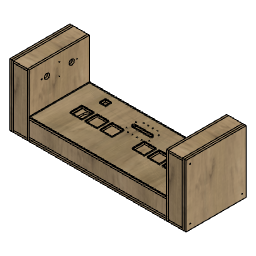
ongekicon-diy (Autodesk Fusion 360 design; units mm, degrees)
Autodesk Fusion 360 part; units mm, degrees
sketch "스케치1" plane through (0, 0, 0) normal (0, 0, 1) x (1, 0, 0)
  line L0 (289, -642.7336) -> (375, -642.7336)
  line L1 (375, -656.7336) -> (289, -656.7336)
  arc A0 (289, -642.7336) -> (289, -656.7336) centre (289, -649.7336) ccw
  arc A1 (375, -656.7336) -> (375, -642.7336) centre (375, -649.7336) ccw
  arc A2 (375, -656.7336) -> (375, -642.7336) centre (375, -649.7336) ccw
  circle A3 centre (277.0783, -626.5501) radius 2.65
  circle A4 centre (277.0783, -672.9171) radius 2.65
  circle A5 centre (386.9217, -626.4866) radius 2.65
  circle A6 centre (386.9217, -672.8535) radius 2.65
  circle A7 centre (299.0783, -611.6097) radius 2.65
  circle A8 centre (321.0783, -611.6097) radius 2.65
  circle A9 centre (343.0783, -611.6097) radius 2.65
  circle A10 centre (365.0783, -611.6097) radius 2.65
  circle A11 centre (364.9217, -687.7939) radius 2.65
  circle A12 centre (342.9217, -687.7939) radius 2.65
  circle A13 centre (320.9217, -687.7939) radius 2.65
  circle A14 centre (298.9217, -687.7939) radius 2.65
  line L2 (0, -575) -> (664, -575)
  line L3 (664, -575) -> (664, -866)
  line L4 (664, -866) -> (0, -866)
  line L5 (0, -866) -> (0, -575)
  line L6 (0, -1260) -> (664, -1260)
  line L7 (664, -1260) -> (664, -1333)
  line L8 (664, -1333) -> (0, -1333)
  line L9 (0, -1333) -> (0, -1260)
  line L10 (0, -1495) -> (0, -1422)
  line L11 (664, -1422) -> (664, -1495)
  line L12 (0, -1422) -> (664, -1422)
  line L13 (664, -1495) -> (0, -1495)
  line L14 (664, 150) -> (664, -141)
  line L15 (0, -141) -> (0, 150)
  line L16 (664, -141) -> (0, -141)
  line L17 (604, 120) -> (60, 120)
  line L18 (634, -81) -> (634, 90)
  line L19 (30, 90) -> (30, -81)
  line L20 (60, -111) -> (604, -111)
  line L21 (0, 150) -> (664, 150)
  line L22 (634, -431) -> (634, -260)
  line L23 (664, -200) -> (664, -491)
  line L24 (0, -200) -> (664, -200)
  line L25 (60, -461) -> (604, -461)
  line L26 (664, -491) -> (0, -491)
  line L27 (30, -260) -> (30, -431)
  line L28 (604, -230) -> (60, -230)
  line L29 (0, -491) -> (0, -200)
  line L30 (0, -230) -> (0, -200) construction
  arc A15 (60, 120) -> (30, 90) centre (60, 90) ccw
  arc A16 (634, 90) -> (604, 120) centre (604, 90) ccw
  arc A17 (604, -111) -> (634, -81) centre (604, -81) ccw
  arc A18 (30, -81) -> (60, -111) centre (60, -81) ccw
  arc A19 (60, -230) -> (30, -260) centre (60, -260) ccw
  arc A20 (634, -260) -> (604, -230) centre (604, -260) ccw
  arc A21 (604, -461) -> (634, -431) centre (604, -431) ccw
  arc A22 (30, -431) -> (60, -461) centre (60, -431) ccw
  circle A23 centre (644.0002, -219.9998) radius 3.25
  circle A24 centre (644.0002, -471.0002) radius 3.25
  circle A25 centre (644.0002, -121.0002) radius 9
  circle A26 centre (644.0002, 130.0002) radius 9
  circle A27 centre (19.9998, 130.0002) radius 9
  circle A28 centre (19.9998, -121.0002) radius 9
  circle A29 centre (19.9998, -219.9998) radius 3.25
  circle A30 centre (19.9998, -471.0002) radius 3.25
  line L31 (1066.4968, -1645.2647) -> (1357.4968, -1645.2647)
  line L32 (1357.4968, -1645.2647) -> (1357.4968, -1712.2647)
  line L33 (1357.4968, -1712.2647) -> (1066.4968, -1712.2647)
  line L34 (1066.4968, -1712.2647) -> (1066.4968, -1645.2647)
  line L35 (716.4968, -1645.2647) -> (1007.4968, -1645.2647)
  line L36 (1007.4968, -1645.2647) -> (1007.4968, -1712.2647)
  line L37 (1007.4968, -1712.2647) -> (716.4968, -1712.2647)
  line L38 (716.4968, -1712.2647) -> (716.4968, -1645.2647)
  line L39 (1066.4968, -845.2647) -> (1357.4968, -845.2647)
  line L40 (1357.4968, -845.2647) -> (1357.4968, -912.2647)
  line L41 (1357.4968, -912.2647) -> (1066.4968, -912.2647)
  line L42 (1066.4968, -912.2647) -> (1066.4968, -845.2647)
  line L43 (716.4968, -845.2647) -> (1007.4968, -845.2647)
  line L44 (1007.4968, -845.2647) -> (1007.4968, -912.2647)
  line L45 (1007.4968, -912.2647) -> (716.4968, -912.2647)
  line L46 (716.4968, -912.2647) -> (716.4968, -845.2647)
  line L47 (1406.0943, -1345.433) -> (1473.0943, -1345.433)
  line L48 (1473.0943, -1345.433) -> (1473.0943, -1627.433)
  line L49 (1473.0943, -1627.433) -> (1406.0943, -1627.433)
  line L50 (1406.0943, -1627.433) -> (1406.0943, -1345.433)
  line L51 (1573.0943, -1627.433) -> (1506.0943, -1627.433)
  line L52 (1506.0943, -1627.433) -> (1506.0943, -1345.433)
  line L53 (1506.0943, -1345.433) -> (1573.0943, -1345.433)
  line L54 (1573.0943, -1345.433) -> (1573.0943, -1627.433)
  line L55 (1506.0943, -1277.433) -> (1506.0943, -995.433)
  line L56 (1506.0943, -995.433) -> (1573.0943, -995.433)
  line L57 (1573.0943, -995.433) -> (1573.0943, -1277.433)
  line L58 (1573.0943, -1277.433) -> (1506.0943, -1277.433)
  line L59 (1406.0943, -1277.433) -> (1406.0943, -995.433)
  line L60 (1406.0943, -995.433) -> (1473.0943, -995.433)
  line L61 (1473.0943, -1277.433) -> (1406.0943, -1277.433)
  line L62 (1473.0943, -995.433) -> (1473.0943, -1277.433)
  line L63 (725.4968, -1278.433) -> (716.4968, -1278.433)
  line L64 (998.4968, -1278.433) -> (725.4968, -1278.433)
  line L65 (998.4968, -1278.433) -> (1007.4968, -1278.433)
  line L66 (1007.4968, -978.433) -> (1007.4968, -1278.433)
  line L67 (1007.4968, -978.433) -> (716.4968, -978.433)
  line L68 (716.4968, -978.433) -> (716.4968, -1278.433)
  arc A31 (1661.5009, -1535.9592) -> (1691.5009, -1565.9592) centre (1691.5009, -1535.9592) ccw
  line L69 (1871.5009, -1325.9592) -> (1691.5009, -1325.9592)
  arc A32 (1691.5009, -1325.9592) -> (1661.5009, -1355.9592) centre (1691.5009, -1355.9592) ccw
  line L70 (1661.5009, -1355.9592) -> (1661.5009, -1535.9592)
  circle A33 centre (1656.0009, -1571.4592) radius 3.25
  circle A34 centre (1656.0009, -1320.4592) radius 3.25
  line L71 (1636.0009, -1295.9592) -> (1636.0009, -1595.9592)
  arc A35 (2251.5009, -1355.9592) -> (2221.5009, -1325.9592) centre (2221.5009, -1355.9592) ccw
  arc A36 (2221.5009, -1565.9592) -> (2251.5009, -1535.9592) centre (2221.5009, -1535.9592) ccw
  circle A37 centre (2257.0009, -1571.4592) radius 10
  circle A38 centre (2257.0009, -1320.4592) radius 10
  circle A39 centre (2006.0009, -1571.4592) radius 10
  line L72 (2221.5009, -1325.9592) -> (2041.5009, -1325.9592)
  circle A40 centre (2006.0009, -1320.4592) radius 10
  line L73 (2041.5009, -1565.9592) -> (2221.5009, -1565.9592)
  line L74 (2277.0009, -1295.9592) -> (2277.0009, -1595.9592)
  arc A41 (2011.5009, -1535.9592) -> (2041.5009, -1565.9592) centre (2041.5009, -1535.9592) ccw
  arc A42 (2041.5009, -1325.9592) -> (2011.5009, -1355.9592) centre (2041.5009, -1355.9592) ccw
  line L75 (2251.5009, -1535.9592) -> (2251.5009, -1355.9592)
  line L76 (2011.5009, -1355.9592) -> (2011.5009, -1535.9592)
  line L77 (1986.0009, -1295.9592) -> (1986.0009, -1595.9592)
  line L78 (1927.0009, -1295.9592) -> (1927.0009, -1595.9592)
  line L79 (1901.5009, -1535.9592) -> (1901.5009, -1355.9592)
  line L80 (1691.5009, -1565.9592) -> (1871.5009, -1565.9592)
  arc A43 (1871.5009, -1565.9592) -> (1901.5009, -1535.9592) centre (1871.5009, -1535.9592) ccw
  arc A44 (1901.5009, -1355.9592) -> (1871.5009, -1325.9592) centre (1871.5009, -1355.9592) ccw
  circle A45 centre (1907.0009, -1320.4592) radius 3.25
  circle A46 centre (1907.0009, -1571.4592) radius 3.25
  line L81 (1927.0009, -1295.9592) -> (1636.0009, -1295.9592)
  line L82 (1927.0009, -1595.9592) -> (1636.0009, -1595.9592)
  line L83 (2277.0009, -1595.9592) -> (1986.0009, -1595.9592)
  line L84 (2277.0009, -1295.9592) -> (1986.0009, -1295.9592)
  line L85 (1927.0009, -1245.9592) -> (1636.0009, -1245.9592)
  line L86 (1927.0009, -945.9592) -> (1927.0009, -1245.9592)
  line L87 (1661.5009, -1005.9592) -> (1661.5009, -1185.9592)
  line L88 (1636.0009, -945.9592) -> (1636.0009, -1245.9592)
  arc A47 (1901.5009, -1005.9592) -> (1871.5009, -975.9592) centre (1871.5009, -1005.9592) ccw
  circle A48 centre (1907.0009, -1221.4592) radius 3.25
  circle A49 centre (1656.0009, -970.4592) radius 3.25
  circle A50 centre (1907.0009, -970.4592) radius 3.25
  line L89 (2277.0009, -945.9592) -> (2277.0009, -1245.9592)
  line L90 (2041.5009, -1215.9592) -> (2221.5009, -1215.9592)
  line L91 (2277.0009, -945.9592) -> (1986.0009, -945.9592)
  line L92 (1691.5009, -1215.9592) -> (1871.5009, -1215.9592)
  line L93 (1901.5009, -1185.9592) -> (1901.5009, -1005.9592)
  arc A51 (1871.5009, -1215.9592) -> (1901.5009, -1185.9592) centre (1871.5009, -1185.9592) ccw
  line L94 (1871.5009, -975.9592) -> (1691.5009, -975.9592)
  line L95 (1986.0009, -945.9592) -> (1986.0009, -1245.9592)
  circle A52 centre (1656.0009, -1221.4592) radius 3.25
  arc A53 (1661.5009, -1185.9592) -> (1691.5009, -1215.9592) centre (1691.5009, -1185.9592) ccw
  arc A54 (1691.5009, -975.9592) -> (1661.5009, -1005.9592) centre (1691.5009, -1005.9592) ccw
  line L96 (1927.0009, -945.9592) -> (1636.0009, -945.9592)
  arc A55 (2011.5009, -1185.9592) -> (2041.5009, -1215.9592) centre (2041.5009, -1185.9592) ccw
  circle A56 centre (2257.0009, -970.4592) radius 10
  circle A57 centre (2006.0009, -1221.4592) radius 10
  line L97 (2011.5009, -1005.9592) -> (2011.5009, -1185.9592)
  arc A58 (2041.5009, -975.9592) -> (2011.5009, -1005.9592) centre (2041.5009, -1005.9592) ccw
  circle A59 centre (2257.0009, -1221.4592) radius 10
  circle A60 centre (2006.0009, -970.4592) radius 10
  line L98 (2277.0009, -1245.9592) -> (1986.0009, -1245.9592)
  line L99 (2251.5009, -1185.9592) -> (2251.5009, -1005.9592)
  arc A61 (2221.5009, -1215.9592) -> (2251.5009, -1185.9592) centre (2221.5009, -1185.9592) ccw
  line L100 (2221.5009, -975.9592) -> (2041.5009, -975.9592)
  arc A62 (2251.5009, -1005.9592) -> (2221.5009, -975.9592) centre (2221.5009, -1005.9592) ccw
  line L101 (716.4968, -1317.433) -> (716.4968, -1617.433)
  circle A63 centre (801.9968, -1386.933) radius 12.5
  line L102 (1007.4968, -1317.433) -> (716.4968, -1317.433)
  line L103 (1007.4968, -1617.433) -> (716.4968, -1617.433)
  circle A64 centre (921.9968, -1386.933) radius 12.5
  line L104 (716.4968, -1521.933) -> (716.4968, -1617.433)
  circle A65 centre (946.9968, -1386.933) radius 2.2361
  circle A66 centre (776.9968, -1386.933) radius 2.2592
  circle A67 centre (861.9968, -1416.933) radius 2.2361
  line L105 (1007.4968, -1317.433) -> (1007.4968, -1617.433)
  circle A68 centre (861.9968, -1356.933) radius 2.2361
  circle A69 centre (736.4968, -1253.933) radius 2.5
  circle A70 centre (987.4968, -1253.933) radius 2.5
  circle A71 centre (987.4968, -1002.933) radius 2.5
  circle A72 centre (1086.4968, -1002.933) radius 2.5
  line L106 (1066.4968, -978.433) -> (1066.4968, -1278.433)
  circle A73 centre (1086.4968, -1253.933) radius 2.5
  line L107 (1348.4968, -1278.433) -> (1357.4968, -1278.433)
  line L108 (1348.4968, -1278.433) -> (1075.4968, -1278.433)
  line L109 (1357.4968, -978.433) -> (1066.4968, -978.433)
  line L110 (1357.4968, -978.433) -> (1357.4968, -1278.433)
  line L111 (1075.4968, -1278.433) -> (1066.4968, -1278.433)
  circle A74 centre (1337.4968, -1253.933) radius 2.5
  circle A75 centre (1337.4968, -1002.933) radius 2.5
  circle A76 centre (456.3298, -1576.2079) radius 4
  circle A77 centre (547.3298, -1605.2079) radius 4
  circle A78 centre (592.8298, -1590.7079) radius 4
  circle A79 centre (547.3298, -1576.2079) radius 4
  circle A80 centre (410.8298, -1590.7079) radius 4
  circle A81 centre (501.8298, -1590.7079) radius 4
  circle A82 centre (456.3298, -1605.2079) radius 4
  line L112 (521.8298, -1571.2079) -> (481.2298, -1571.2079)
  line L113 (479.3298, -1573.1079) -> (479.3298, -1578.7079)
  line L114 (481.8298, -1581.2079) -> (521.8298, -1581.2079)
  line L115 (524.3298, -1578.7079) -> (524.3298, -1573.7079)
  arc A83 (524.3298, -1573.7079) -> (521.8298, -1571.2079) centre (521.8298, -1573.7079) ccw
  arc A84 (521.8298, -1581.2079) -> (524.3298, -1578.7079) centre (521.8298, -1578.7079) ccw
  arc A85 (479.3298, -1578.7079) -> (481.8298, -1581.2079) centre (481.8298, -1578.7079) ccw
  arc A86 (481.2298, -1571.2079) -> (479.3298, -1573.1079) centre (481.2298, -1573.1079) ccw
  line L116 (365.3298, -1554.2079) -> (638.3298, -1554.2079)
  line L117 (638.3298, -1554.2079) -> (638.3298, -1627.2079)
  line L118 (638.3298, -1627.2079) -> (365.3298, -1627.2079)
  line L119 (365.3298, -1627.2079) -> (365.3298, -1554.2079)
  arc A87 (884.4968, -1545.933) -> (881.9968, -1543.433) centre (881.9968, -1545.933) ccw
  line L120 (884.4968, -1550.933) -> (884.4968, -1545.933)
  line L121 (881.9968, -1543.433) -> (841.3968, -1543.433)
  arc A88 (881.9968, -1553.433) -> (884.4968, -1550.933) centre (881.9968, -1550.933) ccw
  arc A89 (839.4968, -1550.933) -> (841.9968, -1553.433) centre (841.9968, -1550.933) ccw
  circle A90 centre (816.4968, -1577.433) radius 4
  circle A91 centre (861.9968, -1562.933) radius 4
  line L122 (841.9968, -1553.433) -> (881.9968, -1553.433)
  arc A92 (841.3968, -1543.433) -> (839.4968, -1545.333) centre (841.3968, -1545.333) ccw
  circle A93 centre (816.4968, -1548.433) radius 4
  line L123 (839.4968, -1545.333) -> (839.4968, -1550.933)
  circle A94 centre (770.9968, -1562.933) radius 4
  circle A95 centre (952.9968, -1562.933) radius 4
  circle A96 centre (907.4968, -1577.433) radius 4
  circle A97 centre (907.4968, -1548.433) radius 4
  circle A98 centre (1302.9968, -1562.933) radius 4
  circle A99 centre (1257.4968, -1548.433) radius 4
  arc A100 (1231.9968, -1553.433) -> (1234.4968, -1550.933) centre (1231.9968, -1550.933) ccw
  arc A101 (1234.4968, -1545.933) -> (1231.9968, -1543.433) centre (1231.9968, -1545.933) ccw
  line L124 (1231.9968, -1543.433) -> (1191.3968, -1543.433)
  circle A102 centre (1211.9968, -1562.933) radius 4
  circle A103 centre (1257.4968, -1577.433) radius 4
  line L125 (1357.4968, -1317.433) -> (1357.4968, -1617.433)
  arc A104 (1189.4968, -1550.933) -> (1191.9968, -1553.433) centre (1191.9968, -1550.933) ccw
  circle A105 centre (1120.9968, -1562.933) radius 4
  line L126 (1234.4968, -1550.933) -> (1234.4968, -1545.933)
  circle A106 centre (1211.9968, -1356.933) radius 2.2361
  circle A107 centre (1166.4968, -1548.433) radius 4
  arc A108 (1191.3968, -1543.433) -> (1189.4968, -1545.333) centre (1191.3968, -1545.333) ccw
  line L127 (1189.4968, -1545.333) -> (1189.4968, -1550.933)
  circle A109 centre (1166.4968, -1577.433) radius 4
  circle A110 centre (1211.9968, -1416.933) radius 2.2361
  circle A111 centre (1126.9968, -1386.933) radius 2.2592
  line L128 (1191.9968, -1553.433) -> (1231.9968, -1553.433)
  circle A112 centre (1151.9968, -1386.933) radius 12.5
  line L129 (1357.4968, -1617.433) -> (1066.4968, -1617.433)
  line L130 (1066.4968, -1521.933) -> (1066.4968, -1617.433)
  line L131 (1066.4968, -1317.433) -> (1066.4968, -1617.433)
  line L132 (1357.4968, -1317.433) -> (1066.4968, -1317.433)
  circle A113 centre (1296.9968, -1386.933) radius 2.2361
  circle A114 centre (1271.9968, -1386.933) radius 12.5
  line L133 (121.8298, -1581.2079) -> (161.8298, -1581.2079)
  line L134 (161.8298, -1571.2079) -> (121.2298, -1571.2079)
  line L135 (119.3298, -1573.1079) -> (119.3298, -1578.7079)
  line L136 (278.3298, -1554.2079) -> (278.3298, -1627.2079)
  arc A115 (161.8298, -1581.2079) -> (164.3298, -1578.7079) centre (161.8298, -1578.7079) ccw
  arc A116 (119.3298, -1578.7079) -> (121.8298, -1581.2079) centre (121.8298, -1578.7079) ccw
  circle A117 centre (187.3298, -1576.2079) radius 4
  arc A118 (121.2298, -1571.2079) -> (119.3298, -1573.1079) centre (121.2298, -1573.1079) ccw
  line L137 (164.3298, -1578.7079) -> (164.3298, -1573.7079)
  circle A119 centre (187.3298, -1605.2079) radius 4
  circle A120 centre (141.8298, -1590.7079) radius 4
  arc A121 (164.3298, -1573.7079) -> (161.8298, -1571.2079) centre (161.8298, -1573.7079) ccw
  line L138 (278.3298, -1627.2079) -> (5.3298, -1627.2079)
  circle A122 centre (96.3298, -1576.2079) radius 4
  circle A123 centre (232.8298, -1590.7079) radius 4
  line L139 (5.3298, -1627.2079) -> (5.3298, -1554.2079)
  circle A124 centre (50.8298, -1590.7079) radius 4
  circle A125 centre (96.3298, -1605.2079) radius 4
  line L140 (5.3298, -1554.2079) -> (278.3298, -1554.2079)
  line L141 (138.1898, -635.6975) -> (109.1898, -635.6975)
  line L142 (109.1898, -635.6975) -> (109.1898, -606.6975)
  line L143 (109.1898, -606.6975) -> (138.1898, -606.6975)
  line L144 (138.1898, -606.6975) -> (138.1898, -635.6975)
  line L145 (525.8102, -635.6975) -> (554.8102, -635.6975)
  line L146 (554.8102, -635.6975) -> (554.8102, -606.6975)
  line L147 (554.8102, -606.6975) -> (525.8102, -606.6975)
  line L148 (525.8102, -606.6975) -> (525.8102, -635.6975)
  line L149 (554.8102, -985.6975) -> (554.8102, -956.6975)
  line L150 (109.1898, -985.6975) -> (109.1898, -956.6975)
  line L151 (138.1898, -956.6975) -> (138.1898, -985.6975)
  line L152 (525.8102, -956.6975) -> (525.8102, -985.6975)
  line L153 (525.8102, -985.6975) -> (554.8102, -985.6975)
  line L154 (664, -925) -> (664, -1216)
  line L155 (0, -1216) -> (0, -925)
  line L156 (109.1898, -956.6975) -> (138.1898, -956.6975)
  arc A126 (289, -992.7336) -> (289, -1006.7336) centre (289, -999.7336) ccw
  arc A127 (375, -1006.7336) -> (375, -992.7336) centre (375, -999.7336) ccw
  arc A128 (375, -1006.7336) -> (375, -992.7336) centre (375, -999.7336) ccw
  line L157 (138.1898, -985.6975) -> (109.1898, -985.6975)
  line L158 (375, -1006.7336) -> (289, -1006.7336)
  line L159 (664, -1216) -> (0, -1216)
  line L160 (0, -925) -> (664, -925)
  line L161 (289, -992.7336) -> (375, -992.7336)
  line L162 (554.8102, -956.6975) -> (525.8102, -956.6975)
  circle A129 centre (644, 254) radius 2.5
  circle A130 centre (644, 505) radius 2.5
  line L163 (664, 525) -> (664, 234)
  line L164 (0, 525) -> (664, 525)
  line L165 (664, 234) -> (0, 234)
  line L166 (0, 234) -> (0, 525)
  circle A131 centre (20, 254) radius 2.5
  circle A132 centre (20, 505) radius 2.5
  line L167 (180.5, -1312) -> (151.5, -1312)
  line L168 (151.5, -1312) -> (151.5, -1283)
  line L169 (151.5, -1283) -> (180.5, -1283)
  line L170 (180.5, -1283) -> (180.5, -1312)
  line L171 (318.75, -1303.75) -> (306.25, -1303.75)
  line L172 (306.25, -1303.75) -> (306.25, -1291.25)
  line L173 (306.25, -1291.25) -> (318.75, -1291.25)
  line L174 (318.75, -1291.25) -> (318.75, -1303.75)
  line L175 (483.5, -1312) -> (512.5, -1312)
  line L176 (512.5, -1312) -> (512.5, -1283)
  line L177 (483.5, -1283) -> (483.5, -1312)
  line L178 (512.5, -1283) -> (483.5, -1283)
  line L179 (357.75, -1303.75) -> (357.75, -1291.25)
  line L180 (357.75, -1291.25) -> (345.25, -1291.25)
  line L181 (345.25, -1303.75) -> (357.75, -1303.75)
  line L182 (345.25, -1291.25) -> (345.25, -1303.75)
  line L183 (136.915, -748.0793) -> (78.915, -748.0793)
  line L184 (78.915, -748.0793) -> (78.915, -690.0793)
  line L185 (78.915, -690.0793) -> (136.915, -690.0793)
  line L186 (136.915, -690.0793) -> (136.915, -748.0793)
  line L187 (209.8081, -748.0793) -> (151.8081, -748.0793)
  line L188 (151.8081, -748.0793) -> (151.8081, -690.0793)
  line L189 (151.8081, -690.0793) -> (209.8081, -690.0793)
  line L190 (209.8081, -690.0793) -> (209.8081, -748.0793)
  line L191 (282.7013, -748.0793) -> (224.7013, -748.0793)
  line L192 (224.7013, -748.0793) -> (224.7013, -690.0793)
  line L193 (224.7013, -690.0793) -> (282.7013, -690.0793)
  line L194 (282.7013, -690.0793) -> (282.7013, -748.0793)
  line L195 (512.1919, -690.0793) -> (454.1919, -690.0793)
  line L196 (527.085, -748.0793) -> (585.085, -748.0793)
  line L197 (454.1919, -748.0793) -> (512.1919, -748.0793)
  line L198 (585.085, -748.0793) -> (585.085, -690.0793)
  line L199 (381.2987, -690.0793) -> (381.2987, -748.0793)
  line L200 (381.2987, -748.0793) -> (439.2987, -748.0793)
  line L201 (454.1919, -690.0793) -> (454.1919, -748.0793)
  line L202 (585.085, -690.0793) -> (527.085, -690.0793)
  line L203 (439.2987, -690.0793) -> (381.2987, -690.0793)
  line L204 (527.085, -690.0793) -> (527.085, -748.0793)
  line L205 (512.1919, -748.0793) -> (512.1919, -690.0793)
  line L206 (439.2987, -748.0793) -> (439.2987, -690.0793)
  line L207 (152.5581, -1098.8293) -> (152.5581, -1040.8293)
  line L208 (79.665, -1098.8293) -> (79.665, -1040.8293)
  line L209 (79.665, -1040.8293) -> (137.665, -1040.8293)
  line L210 (152.5581, -1040.8293) -> (210.5581, -1040.8293)
  line L211 (137.665, -1040.8293) -> (137.665, -1098.8293)
  line L212 (210.5581, -1098.8293) -> (152.5581, -1098.8293)
  line L213 (137.665, -1098.8293) -> (79.665, -1098.8293)
  line L214 (210.5581, -1040.8293) -> (210.5581, -1098.8293)
  line L215 (225.4513, -1098.8293) -> (225.4513, -1040.8293)
  line L216 (283.4513, -1098.8293) -> (225.4513, -1098.8293)
  line L217 (225.4513, -1040.8293) -> (283.4513, -1040.8293)
  line L218 (283.4513, -1040.8293) -> (283.4513, -1098.8293)
  line L219 (526.335, -1098.8293) -> (584.335, -1098.8293)
  line L220 (526.335, -1040.8293) -> (526.335, -1098.8293)
  line L221 (380.5487, -1040.8293) -> (380.5487, -1098.8293)
  line L222 (380.5487, -1098.8293) -> (438.5487, -1098.8293)
  line L223 (453.4419, -1040.8293) -> (453.4419, -1098.8293)
  line L224 (438.5487, -1098.8293) -> (438.5487, -1040.8293)
  line L225 (438.5487, -1040.8293) -> (380.5487, -1040.8293)
  line L226 (511.4419, -1098.8293) -> (511.4419, -1040.8293)
  line L227 (453.4419, -1098.8293) -> (511.4419, -1098.8293)
  line L228 (584.335, -1098.8293) -> (584.335, -1040.8293)
  line L229 (511.4419, -1040.8293) -> (453.4419, -1040.8293)
  line L230 (584.335, -1040.8293) -> (526.335, -1040.8293)
  circle A133 centre (736.4968, -1002.933) radius 2.6
  point P0 (0, -350)
  point P1 (2131.5009, -1095.9592)
  point P2 (1781.5009, -1095.9592)
  point P3 (861.9968, -1564.433)
  point P4 (861.9968, -1564.433)
  point P5 (166, -1297.5)
  point P6 (166, -1297.5)
  point P7 (501.8298, -1590.7079)
  point P8 (501.8298, -1576.2079)
  point P9 (861.9968, -1548.433)
  point P10 (861.9968, -1562.933)
  point P11 (1211.9968, -1564.433)
  point P12 (1211.9968, -1548.433)
  point P13 (1211.9968, -1562.933)
  point P14 (1211.9968, -1564.433)
  point P15 (141.8298, -1576.2079)
  point P16 (141.8298, -1590.7079)
  point P17 (540.3102, -621.1975)
  point P18 (253.7013, -719.0793)
  point P19 (107.915, -719.0793)
  point P20 (123.6898, -621.1975)
  point P21 (107.915, -719.0793)
  point P22 (253.7013, -719.0793)
  point P23 (123.6898, -621.1975)
  point P24 (540.3102, -621.1975)
  point P25 (123.6898, -621.1975)
  point P26 (540.3102, -621.1975)
  point P27 (166, -1297.5)
  point P28 (107.915, -719.0793)
  point P29 (180.8081, -719.0793)
  point P30 (253.7013, -719.0793)
  point P31 (556.085, -719.0793)
  point P32 (410.2987, -719.0793)
  point P33 (556.085, -719.0793)
  point P34 (410.2987, -719.0793)
  point P35 (410.2987, -719.0793)
  point P36 (483.1919, -719.0793)
  point P37 (556.085, -719.0793)
  point P38 (79.665, -1040.8293)
  dimension "d11" = 7
  dimension "d22" = 5.3
  dimension "d23" = 5.3
  dimension "d24" = 5.3
  dimension "d25" = 5.3
  dimension "d26" = 5.3
  dimension "d27" = 22
  dimension "d28" = 22
  dimension "d29" = 22
  dimension "d33" = 5.3
  dimension "d34" = 5.3
  dimension "d35" = 5.3
  dimension "d36" = 5.3
  dimension "d37" = 5.3
  dimension "d38" = 5.3
  dimension "d39" = 5.3
  dimension "d43" = 291
  dimension "d64" = 86
  dimension "d194" = 73
  dimension "d195" = 664
  dimension "d196" = 73
  dimension "d350" = 291
  dimension "d357" = 28.284
  dimension "d358" = 28.284
  dimension "d359" = 28.284
  dimension "d360" = 28.284
  dimension "d361" = 664
  dimension "d362" = 291
  dimension "d364" = 28.284
  dimension "d365" = 28.284
  dimension "d366" = 28.284
  dimension "d367" = 28.284
  dimension "d368" = 30
  dimension "d369" = 30
  dimension "d370" = 30
  dimension "d371" = 30
  dimension "d372" = 30
  dimension "d373" = 30
  dimension "d374" = 30
  dimension "d375" = 30
  dimension "d376" = 6.5
  dimension "d377" = 6.5
  dimension "d378" = 18
  dimension "d379" = 18
  dimension "d380" = 18
  dimension "d381" = 18
  dimension "d382" = 6.5
  dimension "d383" = 6.5
  dimension "d537" = 664
  dimension "d553" = 67
  dimension "d554" = 67
  dimension "d555" = 67
  dimension "d556" = 67
  dimension "d807" = 300
  dimension "d858" = 30
  dimension "d859" = 30
  dimension "d860" = 30
  dimension "d861" = 30
  dimension "d862" = 6.5
  dimension "d863" = 6.5
  dimension "d865" = 6.5
  dimension "d876" = 30
  dimension "d877" = 30
  dimension "d878" = 30
  dimension "d879" = 30
  dimension "d880" = 20
  dimension "d881" = 20
  dimension "d882" = 20
  dimension "d883" = 20
  dimension "d884" = 6.5
  dimension "d892" = 30
  dimension "d893" = 30
  dimension "d894" = 30
  dimension "d895" = 30
  dimension "d896" = 6.5
  dimension "d897" = 6.5
  dimension "d898" = 6.5
  dimension "d899" = 30
  dimension "d900" = 30
  dimension "d901" = 30
  dimension "d902" = 30
  dimension "d903" = 20
  dimension "d904" = 20
  dimension "d905" = 20
  dimension "d906" = 20
  dimension "d907" = 6.5
  dimension "d934" = 300
  dimension "d943" = 25
  dimension "d944" = 25
  dimension "d954" = 5
  dimension "d955" = 5
  dimension "d956" = 5
  dimension "d957" = 300
  dimension "d966" = 5
  dimension "d967" = 5
  dimension "d968" = 5
  dimension "d969" = 5
  dimension "d1011" = 8
  dimension "d1012" = 8
  dimension "d1013" = 8
  dimension "d1014" = 8
  dimension "d1015" = 8
  dimension "d1016" = 8
  dimension "d1017" = 8
  dimension "d1055" = 2.5
  dimension "d1056" = 1.9
  dimension "d1057" = 273
  dimension "d1058" = 73
  dimension "d1059" = 8
  dimension "d1060" = 8
  dimension "d1061" = 8
  dimension "d1062" = 8
  dimension "d1063" = 8
  dimension "d1064" = 8
  dimension "d1065" = 8
  dimension "d1072" = 2.5
  dimension "d1073" = 1.9
  dimension "d1094" = 25
  dimension "d1095" = 25
  dimension "d1096" = 8
  dimension "d1097" = 8
  dimension "d1098" = 8
  dimension "d1099" = 8
  dimension "d1100" = 8
  dimension "d1101" = 8
  dimension "d1102" = 8
  dimension "d1105" = 2.5
  dimension "d1106" = 1.9
  dimension "d1111" = 8
  dimension "d1112" = 8
  dimension "d1113" = 8
  dimension "d1114" = 8
  dimension "d1115" = 8
  dimension "d1116" = 8
  dimension "d1117" = 8
  dimension "d1124" = 2.5
  dimension "d1125" = 1.9
  dimension "d1126" = 273
  dimension "d1127" = 73
  dimension "d1144" = 29
  dimension "d1145" = 29
  dimension "d1146" = 29
  dimension "d1147" = 29
  dimension "d1148" = 7
  dimension "d1171" = 291
  dimension "d1197" = 664
  dimension "d1210" = 29
  dimension "d1211" = 29
  dimension "d1212" = 29
  dimension "d1213" = 29
  dimension "d1237" = 291
  dimension "d1259" = 5
  dimension "d1260" = 5
  dimension "d1261" = 5
  dimension "d1262" = 5
  dimension "d1263" = 664
  dimension "d1322" = 29
  dimension "d1323" = 29
  dimension "d1324" = 12.5
  dimension "d1325" = 12.5
  dimension "d1326" = 58
  dimension "d1327" = 58
  dimension "d1328" = 58
  dimension "d1329" = 58
  dimension "d1330" = 58
  dimension "d1331" = 58
  dimension "d1335" = 58
  dimension "d1336" = 58
  dimension "d1337" = 58
  dimension "d1338" = 58
  dimension "d1339" = 58
  dimension "d1340" = 58
  dimension "d1347" = 5.2
  constraint horizontal L0
  constraint horizontal L1
  constraint tangent L0 A0
  constraint tangent L1 A0
  constraint tangent L0 A1
  constraint tangent L1 A1
  constraint horizontal L2
  constraint vertical L3
  constraint horizontal L4
  constraint vertical L5
  constraint horizontal L6
  constraint vertical L7
  constraint horizontal L8
  constraint vertical L9
  constraint horizontal L12
  constraint vertical L11
  constraint horizontal L13
  constraint vertical L10
  constraint horizontal L21
  constraint vertical L14
  constraint horizontal L16
  constraint vertical L15
  constraint horizontal L17
  constraint perpendicular L17 L19
  constraint parallel L17 L20
  constraint parallel L18 L19
  constraint horizontal L24
  constraint vertical L23
  constraint horizontal L26
  constraint vertical L29
  constraint horizontal L28
  constraint perpendicular L27 L28
  constraint parallel L25 L28
  constraint parallel L22 L27
  constraint vertical L30
  constraint tangent L17 A15
  constraint tangent L19 A15
  constraint tangent L17 A16
  constraint tangent L18 A16
  constraint tangent L18 A17
  constraint tangent L20 A17
  constraint tangent L19 A18
  constraint tangent L20 A18
  constraint tangent L28 A19
  constraint tangent L27 A19
  constraint tangent L28 A20
  constraint tangent L22 A20
  constraint tangent L22 A21
  constraint tangent L25 A21
  constraint tangent L27 A22
  constraint tangent L25 A22
  constraint horizontal L31
  constraint vertical L32
  constraint horizontal L33
  constraint vertical L34
  constraint horizontal L35
  constraint vertical L36
  constraint horizontal L37
  constraint vertical L38
  constraint horizontal L39
  constraint vertical L40
  constraint horizontal L41
  constraint vertical L42
  constraint horizontal L43
  constraint vertical L44
  constraint horizontal L45
  constraint vertical L46
  constraint horizontal L47
  constraint vertical L48
  constraint horizontal L49
  constraint vertical L50
  constraint horizontal L53
  constraint vertical L54
  constraint horizontal L51
  constraint vertical L52
  constraint horizontal L60
  constraint vertical L62
  constraint horizontal L61
  constraint vertical L59
  constraint horizontal L56
  constraint vertical L57
  constraint horizontal L58
  constraint vertical L55
  constraint vertical L68
  constraint vertical L66
  constraint horizontal L64
  constraint perpendicular L65 L66
  constraint perpendicular L63 L68
  constraint horizontal L67
  constraint vertical L71
  constraint vertical L78
  constraint horizontal L69
  constraint perpendicular L69 L70
  constraint parallel L69 L80
  constraint parallel L70 L79
  constraint tangent L69 A32
  constraint tangent A32 L70
  constraint tangent L69 A44
  constraint tangent L79 A44
  constraint tangent A31 L70
  constraint tangent A31 L80
  constraint tangent L79 A43
  constraint tangent L80 A43
  constraint vertical L77
  constraint vertical L74
  constraint horizontal L72
  constraint perpendicular L72 L76
  constraint parallel L72 L73
  constraint parallel L75 L76
  constraint tangent L72 A42
  constraint tangent A42 L76
  constraint tangent A35 L72
  constraint tangent A35 L75
  constraint tangent A41 L76
  constraint tangent L73 A41
  constraint tangent A36 L75
  constraint tangent A36 L73
  constraint horizontal L81
  constraint horizontal L82
  constraint horizontal L83
  constraint horizontal L84
  constraint vertical L88
  constraint vertical L86
  constraint horizontal L94
  constraint perpendicular L87 L94
  constraint parallel L92 L94
  constraint parallel L87 L93
  constraint tangent L94 A54
  constraint tangent L87 A54
  constraint tangent A47 L94
  constraint tangent A47 L93
  constraint tangent L87 A53
  constraint tangent L92 A53
  constraint tangent L93 A51
  constraint tangent L92 A51
  constraint vertical L95
  constraint vertical L89
  constraint horizontal L100
  constraint perpendicular L97 L100
  constraint parallel L90 L100
  constraint parallel L97 L99
  constraint tangent A58 L100
  constraint tangent L97 A58
  constraint tangent L100 A62
  constraint tangent L99 A62
  constraint tangent A55 L97
  constraint tangent L90 A55
  constraint tangent L99 A61
  constraint tangent L90 A61
  constraint horizontal L96
  constraint horizontal L85
  constraint horizontal L98
  constraint horizontal L91
  constraint vertical L101
  constraint vertical L105
  constraint vertical L104
  constraint horizontal L102
  constraint horizontal L103
  constraint vertical L106
  constraint vertical L110
  constraint horizontal L108
  constraint perpendicular L107 L110
  constraint perpendicular L106 L111
  constraint horizontal L109
  constraint coincident P27 P6
  constraint coincident P7 A81.centre
  constraint horizontal L112
  constraint perpendicular L112 L113
  constraint parallel L112 L114
  constraint parallel L113 L115
  constraint tangent L115 A83
  constraint tangent L112 A83
  constraint tangent L115 A84
  constraint tangent L114 A84
  constraint equal A83 A84
  constraint tangent L113 A85
  constraint tangent L114 A85
  constraint equal A83 A85
  constraint tangent L112 A86
  constraint tangent L113 A86
  constraint horizontal L116
  constraint vertical L117
  constraint horizontal L118
  constraint vertical L119
  constraint coincident P10 A91.centre
  constraint horizontal L121
  constraint perpendicular L121 L123
  constraint parallel L121 L122
  constraint parallel L120 L123
  constraint tangent A87 L120
  constraint tangent A87 L121
  constraint tangent L120 A88
  constraint tangent A88 L122
  constraint equal A87 A88
  constraint tangent A89 L123
  constraint tangent A89 L122
  constraint equal A87 A89
  constraint tangent L121 A92
  constraint tangent A92 L123
  constraint vertical L131
  constraint vertical L125
  constraint vertical L130
  constraint horizontal L132
  constraint horizontal L129
  constraint coincident P13 A102.centre
  constraint horizontal L124
  constraint perpendicular L124 L127
  constraint parallel L124 L128
  constraint parallel L126 L127
  constraint tangent A101 L126
  constraint tangent A101 L124
  constraint tangent A100 L126
  constraint tangent A100 L128
  constraint equal A100 A101
  constraint tangent A104 L127
  constraint tangent A104 L128
  constraint equal A101 A104
  constraint tangent L124 A108
  constraint tangent A108 L127
  constraint coincident P16 A120.centre
  constraint horizontal L134
  constraint perpendicular L134 L135
  constraint parallel L133 L134
  constraint parallel L135 L137
  constraint tangent L137 A121
  constraint tangent L134 A121
  constraint tangent A115 L137
  constraint tangent L133 A115
  constraint equal A115 A121
  constraint tangent L135 A116
  constraint tangent L133 A116
  constraint equal A116 A121
  constraint tangent L134 A118
  constraint tangent L135 A118
  constraint horizontal L140
  constraint vertical L136
  constraint horizontal L138
  constraint vertical L139
  constraint coincident P28 P21
  constraint coincident P30 P22
  constraint coincident P25 P23
  constraint coincident P26 P24
  constraint horizontal L141
  constraint perpendicular L141 L142
  constraint parallel L141 L143
  constraint parallel L142 L144
  constraint horizontal L145
  constraint perpendicular L145 L146
  constraint parallel L145 L147
  constraint parallel L146 L148
  constraint horizontal L161
  constraint horizontal L158
  constraint tangent A126 L161
  constraint tangent A126 L158
  constraint tangent A127 L161
  constraint tangent A127 L158
  constraint horizontal L160
  constraint vertical L154
  constraint horizontal L159
  constraint vertical L155
  constraint horizontal L157
  constraint perpendicular L150 L157
  constraint parallel L156 L157
  constraint parallel L150 L151
  constraint horizontal L153
  constraint perpendicular L149 L153
  constraint parallel L153 L162
  constraint parallel L149 L152
  constraint vertical L163
  constraint horizontal L165
  constraint vertical L166
  constraint horizontal L167
  constraint perpendicular L167 L168
  constraint parallel L167 L169
  constraint parallel L168 L170
  constraint horizontal L171
  constraint perpendicular L171 L172
  constraint parallel L171 L173
  constraint parallel L172 L174
  constraint horizontal L183
  constraint perpendicular L183 L184
  constraint parallel L183 L185
  constraint parallel L184 L186
  constraint horizontal L187
  constraint perpendicular L187 L188
  constraint parallel L187 L189
  constraint parallel L188 L190
  constraint horizontal L191
  constraint perpendicular L191 L192
  constraint parallel L191 L193
  constraint parallel L192 L194
  constraint horizontal L213
  constraint perpendicular L208 L213
  constraint parallel L209 L213
  constraint parallel L208 L211
  constraint horizontal L212
  constraint perpendicular L207 L212
  constraint parallel L210 L212
  constraint parallel L207 L214
  constraint horizontal L216
  constraint perpendicular L215 L216
  constraint parallel L216 L217
  constraint parallel L215 L218
  constraint coincident P38 L208.end
  measures "d11" radius of A0
  measures "d22" diameter of A3
  measures "d23" diameter of A4
  measures "d24" diameter of A5
  measures "d25" diameter of A6
  measures "d26" diameter of A7
  measures "d27" distance of A7.centre A8.centre
  measures "d28" distance of A8.centre A9.centre
  measures "d29" distance of A9.centre A10.centre
  measures "d33" diameter of A8
  measures "d34" diameter of A9
  measures "d35" diameter of A10
  measures "d36" diameter of A11
  measures "d37" diameter of A12
  measures "d38" diameter of A13
  measures "d39" diameter of A14
  measures "d43" distance of L2.start L4.end
  measures "d64" distance of A0.centre A1.centre
  measures "d194" distance of L6.start L8.end
  measures "d195" distance of L11.start L10.end
  measures "d196" distance of L10.start L10.end
  measures "d350" distance of L15.end L15.start
  measures "d357" distance of L14.end A25.centre
  measures "d358" distance of L14.start A26.centre
  measures "d359" distance of L15.end A27.centre
  measures "d360" distance of L15.start A28.centre
  measures "d361" distance of L24.start L23.start
  measures "d362" distance of L24.start L26.end
  measures "d364" distance of L23.end A24.centre
  measures "d365" distance of L23.start A23.centre
  measures "d366" distance of L24.start A29.centre
  measures "d367" distance of L26.end A30.centre
  measures "d368" radius of A15
  measures "d369" radius of A16
  measures "d370" radius of A17
  measures "d371" radius of A18
  measures "d372" radius of A19
  measures "d373" radius of A20
  measures "d374" radius of A21
  measures "d375" radius of A22
  measures "d376" diameter of A23
  measures "d377" diameter of A24
  measures "d378" diameter of A25
  measures "d379" diameter of A26
  measures "d380" diameter of A27
  measures "d381" diameter of A28
  measures "d382" diameter of A29
  measures "d383" diameter of A30
  measures "d537" distance of L2.start L2.end
  measures "d553" distance of L31.start L33.end
  measures "d554" distance of L35.start L37.end
  measures "d555" distance of L39.start L41.end
  measures "d556" distance of L43.start L45.end
  measures "d807" distance of L65.end L66.start
  measures "d858" radius of A32
  measures "d859" radius of A44
  measures "d860" radius of A31
  measures "d861" radius of A43
  measures "d862" diameter of A34
  measures "d863" diameter of A45
  measures "d865" diameter of A33
  measures "d876" radius of A42
  measures "d877" radius of A35
  measures "d878" radius of A41
  measures "d879" radius of A36
  measures "d880" diameter of A40
  measures "d881" diameter of A38
  measures "d882" diameter of A37
  measures "d883" diameter of A39
  measures "d884" diameter of A46
  measures "d892" radius of A54
  measures "d893" radius of A47
  measures "d894" radius of A53
  measures "d895" radius of A51
  measures "d896" diameter of A49
  measures "d897" diameter of A50
  measures "d898" diameter of A52
  measures "d899" radius of A58
  measures "d900" radius of A62
  measures "d901" radius of A55
  measures "d902" radius of A61
  measures "d903" diameter of A60
  measures "d904" diameter of A56
  measures "d905" diameter of A59
  measures "d906" diameter of A57
  measures "d907" diameter of A48
  measures "d934" distance of L74.end L74.start
  measures "d943" diameter of A63
  measures "d944" diameter of A64
  measures "d954" diameter of A69
  measures "d955" diameter of A70
  measures "d956" diameter of A71
  measures "d957" distance of L109.start L107.end
  measures "d966" diameter of A72
  measures "d967" diameter of A73
  measures "d968" diameter of A74
  measures "d969" diameter of A75
  measures "d1011" diameter of A76
  measures "d1012" diameter of A82
  measures "d1013" diameter of A79
  measures "d1014" diameter of A77
  measures "d1015" diameter of A81
  measures "d1016" diameter of A80
  measures "d1017" diameter of A78
  measures "d1055" radius of A83
  measures "d1056" radius of A86
  measures "d1057" distance of L116.start L116.end
  measures "d1058" distance of L116.start L118.end
  measures "d1059" diameter of A93
  measures "d1060" diameter of A90
  measures "d1061" diameter of A97
  measures "d1062" diameter of A96
  measures "d1063" diameter of A91
  measures "d1064" diameter of A94
  measures "d1065" diameter of A95
  measures "d1072" radius of A87
  measures "d1073" radius of A92
  measures "d1094" diameter of A112
  measures "d1095" diameter of A114
  measures "d1096" diameter of A107
  measures "d1097" diameter of A109
  measures "d1098" diameter of A99
  measures "d1099" diameter of A103
  measures "d1100" diameter of A102
  measures "d1101" diameter of A105
  measures "d1102" diameter of A98
  measures "d1105" radius of A101
  measures "d1106" radius of A108
  measures "d1111" diameter of A122
  measures "d1112" diameter of A125
  measures "d1113" diameter of A117
  measures "d1114" diameter of A119
  measures "d1115" diameter of A120
  measures "d1116" diameter of A124
  measures "d1117" diameter of A123
  measures "d1124" radius of A121
  measures "d1125" radius of A118
  measures "d1126" distance of L139.end L136.start
  measures "d1127" distance of L139.end L138.end
  measures "d1144" distance of L142.end L143.end
  measures "d1145" distance of L141.end L142.end
  measures "d1146" distance of L146.end L147.end
  measures "d1147" distance of L145.end L146.end
  measures "d1148" radius of A126
  measures "d1171" distance of L155.start L155.end
  measures "d1197" distance of L154.start L155.end
  measures "d1210" distance of L150.end L151.start
  measures "d1211" distance of L150.end L150.start
  measures "d1212" distance of L152.start L149.end
  measures "d1213" distance of L149.start L149.end
  measures "d1237" distance of L165.end L164.start
  measures "d1259" diameter of A132
  measures "d1260" diameter of A130
  measures "d1261" diameter of A131
  measures "d1262" diameter of A129
  measures "d1263" distance of L163.start L164.start
  measures "d1322" distance of L168.end L169.end
  measures "d1323" distance of L167.end L168.end
  measures "d1324" distance of L172.end L173.end
  measures "d1325" distance of L171.end L172.end
  measures "d1326" distance of L184.end L185.end
  measures "d1327" distance of L183.end L184.end
  measures "d1328" distance of L188.end L189.end
  measures "d1329" distance of L187.end L188.end
  measures "d1330" distance of L192.end L193.end
  measures "d1331" distance of L191.end L192.end
  measures "d1335" distance of P38 L209.end
  measures "d1336" distance of P38 L208.start
  measures "d1337" distance of L210.end L207.end
  measures "d1338" distance of L207.start L207.end
  measures "d1339" distance of L217.end L215.end
  measures "d1340" distance of L215.start L215.end
  measures "d1347" diameter of A133
extrude "돌출62" add sketch "스케치1" along normal blind 5 contours L154 L155 L159 L160 makes body 1
extrude "돌출63" add sketch "스케치1" along normal blind 9 separate body contours L2 L3 L4 L5 | L6 L7 L8 L9 | L10 L11 L12 L13 | L23 L24 L26 L29 | L31 L32 L33 L34 | L35 L36 L37 L38 | L39 L40 L41 L42 | L43 L44 L45 L46 | L47 L48 L49 L50 | L51 L52 L53 L54 | L55 L56 L57 L58 | L59 L60 L61 L62 | L63 L64 L65 L66 L67 L68 | L71 L78 L81 L82 | L85 L86 L88 L96 | L101 L102 L103 L104 L105 | L106 L107 L108 L109 L110 L111 | L116 L117 L118 L119 | L125 L129 L130 L131 L132 | L136 L138 L139 L140 | L163 L164 L165 L166 | A133 makes body 2 at (1528.4276, -1089.433, 0) makes body 3 at (813.4968, -867.598, 0) makes body 4 at (1340.4245, -1498.5046, 0) makes body 5 at (624.4965, -1590.7079, 0) makes body 6 at (435.1019, 338.1172, 0) makes body 7 at (241.3333, -481, 0) makes body 8 at (264.4965, -1590.7079, 0) makes body 9 at (1170.9143, -1087.2127, 0) makes body 10 at (1163.4968, -867.598, 0) makes body 11 at (1550.7609, -1439.433, 0) makes body 12 at (1751.5009, -955.9592, 0) makes body 13 at (1428.4276, -1089.433, 0) makes body 14 at (813.4968, -1667.598, 0) makes body 15 at (990.4245, -1498.5046, 0) makes body 16 at (50.5, -1292, 0) makes body 17 at (348.4329, -826.6931, 0) makes body 18 at (221.3333, -1446.3333, 0) makes body 19 at (813.2197, -1078.1319, 0) makes body 20 at (1163.4968, -1667.598, 0) makes body 21 at (1450.7609, -1439.433, 0) makes body 22 at (1811.5009, -1585.9592, 0)
move_body "정렬110" bodies 7 to x (1, 0, 0) y (0, 1, 0) z (0, 0, 1) at (0, 725, 9)
move_body "이동82" bodies 16 8 5 18 to x (1, 0, 0) y (0, 0, 1) z (0, -1, 0) at (0, -1213.5, 1218.5)
move_body "이동83" bodies 5 8 to x (0, -1, 0) y (1, 0, 0) z (0, 0, 1) at (1446.3298, -980.6702, 0)
move_body "정렬111" bodies 5 to x (1, 0, 0) y (0, 1, 0) z (0, 0, 1) at (431.1702, 1862, 426.7079)
move_body "정렬112" bodies 8 to x (1, 0, 0) y (0, 1, 0) z (0, 0, 1) at (-223.8298, 1502, 426.7079)
move_body "정렬113" bodies 16 to x (1, 0, 0) y (0, 1, 0) z (0, 0, 1) at (0, 1738.5, 132.5)
move_body "정렬114" bodies 18 to x (1, 0, 0) y (0, 1, 0) z (0, 0, 1) at (0, 1456.5, 294.5)
move_body "정렬115" bodies 17 to x (1, 0, 0) y (0, 1, 0) z (0, 0, 1) at (0, 1100, 91)
move_body "정렬116" bodies 1 to x (1, 0, 0) y (0, 1, 0) z (0, 0, 1) at (0, 1450, 100)
move_body "이동84" bodies 3 10 12 20 22 9 4 19 15 14 to x (0, -1, 0) y (1, 0, 0) z (0, 0, 1) at (1628.7615, -195.7679, 0)
move_body "이동85" bodies 12 15 19 4 9 22 to x (0, 0, 1) y (0, 1, 0) z (-1, 0, 0) at (630.3286, 0, -630.3286)
move_body "정렬117" bodies 22 to x (1, 0, 0) y (0, 1, 0) z (0, 0, 1) at (-9, 569.5041, 317.5262)
move_body "정렬118" bodies 10 to x (1, 0, 0) y (0, 1, 0) z (0, 0, 1) at (-171.1683, 0, -280)
move_body "정렬119" bodies 4 to x (1, 0, 0) y (0, 1, 0) z (0, 0, 1) at (-85, 0, 339)
move_body "정렬120" bodies 15 to x (1, 0, 0) y (0, 1, 0) z (0, 0, 1) at (42.6714, 1437.2647, 619)
move_body "정렬121" bodies 14 to x (1, 0, 0) y (0, 1, 0) z (0, 0, 1) at (756.5032, 1437.2647, 0)
move_body "정렬122" bodies 12 to x (1, 0, 0) y (0, 1, 0) z (0, 0, 1) at (118.6714, 2356.7688, 247.5262)
move_body "정렬123" bodies 19 to x (1, 0, 0) y (0, 1, 0) z (0, 0, 1) at (127.6714, 1437.2647, 280)
move_body "정렬124" bodies 20 to x (1, 0, 0) y (0, 1, 0) z (0, 0, 1) at (756.5032, 1787.2647, 291)
move_body "정렬125" bodies 4 to x (1, 0, 0) y (0, 1, 0) z (0, 0, 1) at (-545.3286, 1787.2647, 280)
move_body "정렬126" bodies 10 to x (1, 0, 0) y (0, 1, 0) z (0, 0, 1) at (-621.3286, 1787.2647, 280)
move_body "정렬127" bodies 22 to x (1, 0, 0) y (0, 1, 0) z (0, 0, 1) at (-697.3286, 1787.2647, 280)
move_body "정렬128" bodies 9 to x (1, 0, 0) y (0, 1, 0) z (0, 0, 1) at (-715.3286, 1787.2647, 280)
move_body "정렬129" bodies 3 to x (1, 0, 0) y (0, 1, 0) z (0, 0, 1) at (-792.4968, 1437.2647, 291)
move_body "이동86" bodies 11 13 21 2 to x (1, 0, 0) y (0, 0, 1) z (0, -1, 0) at (0, -1481.933, 1490.933)
move_body "정렬130" bodies 21 to x (1, 0, 0) y (0, 1, 0) z (0, 0, 1) at (-733.0943, 1724.933, 145.5)
move_body "정렬131" bodies 11 to x (1, 0, 0) y (0, 1, 0) z (0, 0, 1) at (-833.0943, 2006.933, 145.5)
move_body "정렬132" bodies 2 to x (1, 0, 0) y (0, 1, 0) z (0, 0, 1) at (-1582.0943, 2006.933, -204.5)
move_body "정렬133" bodies 13 to x (1, 0, 0) y (0, 1, 0) z (0, 0, 1) at (-1482.0943, 1724.933, -204.5)
